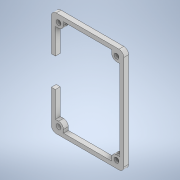
# Autodesk Inventor part: level1_up
Saved by Autodesk Inventor 2021.2 (Build 252289000, 289)
## iProperties
Created: 2021-11-19
Part Number: level1_up
Material: Типовые
Document SubType Name: Modeling
Designer: kanad
Density: 1 g/cm^3
Appearance: По умолчанию
Author: kanad
Autodesk Inventor part; units mm, degrees
ref_plane "YZ Plane" through (0, 0, 0) normal (1, 0, 0) x (0, 1, 0)
ref_plane "XZ Plane" through (0, 0, 0) normal (0, 1, 0) x (-1, 0, 0)
ref_plane "XY Plane" through (0, 0, 0) normal (0, 0, 1) x (1, 0, 0)
sketch "Эскиз1" plane through (0, 0, 0) normal (0, 0, 1) x (1, 0, 0)
  line L0 (19.5, 32.5) -> (-19.5, 32.5)
  line L1 (-22.5, 29.5) -> (-22.5, -29.5)
  line L2 (-19.5, -32.5) -> (19.5, -32.5)
  line L3 (22.5, -29.5) -> (22.5, 29.5)
  line L4 (22.5, 32.5) -> (-22.5, -32.5) construction
  line L5 (-22.5, 32.5) -> (22.5, -32.5) construction
  circle A0 centre (18, 28) radius 1.5 projected
  circle A1 centre (18, -28) radius 1.5 projected
  circle A2 centre (-18, -28) radius 1.5 projected
  circle A3 centre (-18, 28) radius 1.5 projected
  arc A4 (22.5, 29.5) -> (19.5, 32.5) centre (19.5, 29.5) ccw
  arc A5 (19.5, -32.5) -> (22.5, -29.5) centre (19.5, -29.5) ccw
  arc A6 (-22.5, -29.5) -> (-19.5, -32.5) centre (-19.5, -29.5) ccw
  arc A7 (-19.5, 32.5) -> (-22.5, 29.5) centre (-19.5, 29.5) ccw
  line L6 (20, -30) -> (20, 30) projected
  line L7 (20, 30) -> (-20, 30) projected
  line L8 (-20, 30) -> (-20, 9) projected
  line L9 (-20, -9) -> (-20, -30) projected
  line L10 (-20, -30) -> (20, -30) projected
  line L11 (20, -30) -> (15, -30)
  line L12 (15, -30) -> (15, -28)
  line L13 (18, -25) -> (20, -25)
  line L14 (20, -25) -> (20, -30)
  arc A8 (18, -25) -> (15, -28) centre (18, -28) ccw
  line L15 (20, 30) -> (15, 30)
  line L16 (15, 30) -> (15, 28)
  line L17 (18, 25) -> (20, 25)
  line L18 (20, 25) -> (20, 30)
  line L19 (-20, 30) -> (-15, 30)
  line L20 (-15, 30) -> (-15, 28)
  line L21 (-18, 25) -> (-20, 25)
  line L22 (-20, 25) -> (-20, 30)
  line L23 (-20, -30) -> (-15, -30)
  line L24 (-15, -30) -> (-15, -28)
  line L25 (-18, -25) -> (-20, -25)
  line L26 (-20, -25) -> (-20, -30)
  arc A9 (15, 28) -> (18, 25) centre (18, 28) ccw
  arc A10 (-18, 25) -> (-15, 28) centre (-18, 28) ccw
  arc A11 (-15, -28) -> (-18, -25) centre (-18, -28) ccw
  line L27 (-20, 9) -> (-22.5, 9)
  line L28 (-20, -9) -> (-22.5, -9)
  point P0 (0, 0)
  point P1 (15, -25)
  point P2 (15, 25)
  point P3 (-15, 25)
  point P4 (-15, -25)
  dimension "d0" = 45
  dimension "d1" = 65
  dimension "d2" = 3
  dimension "d3" = 5
  dimension "d4" = 5
  dimension "d5" = 3
  dimension "d6" = 5
  dimension "d7" = 5
  dimension "d8" = 5
  dimension "d9" = 5
  dimension "d10" = 5
  dimension "d11" = 3
  constraints: 48 end point, 18 point on line, 16 point on circle, 16 tangent, 11 parallel, 8 centre point, 6 horizontal, 5 equal radius, 5 perpendicular, 2 midpoint
  measures "d0" distance of L5.end L4.end
  measures "d1" distance of L4.end L5.start
  measures "d2" radius of A4
  measures "d3" distance of point (15, -25) L13.end
  measures "d4" distance of L11.end point (15, -25)
  measures "d5" radius of A8
  measures "d6" distance of point (15, 25) L15.end
  measures "d7" distance of point (-15, 25) L21.end
  measures "d8" distance of L19.end point (-15, 25)
  measures "d9" distance of L25.end point (-15, -25)
  measures "d10" distance of point (-15, -25) L23.end
  measures "d11" radius of A9
extrude "Выдавливание1" add sketch "Эскиз1" along normal blind 3 contours A4 L3 A5 L2 A6 L1 L28 L9 L10 L6 L7 L8 L27 A7 L0 | L8 L7 L20 A10 L21 | L25 A11 L24 L10 L9 | L7 L6 L17 A9 L16 | L12 A8 L13 L6 L10
